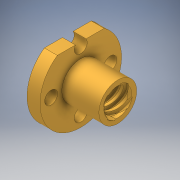
# Autodesk Inventor part: T8_Lead_Screw_Nut
Saved by Autodesk Inventor 2020.3 (Build 243373000, 373)
## iProperties
Created: 2020-06-14
Part Number: T8_Lead_Screw_Nut
Material: Brass, Soft Yellow
Document SubType Name: Modeling
Designer: rah75
Density: 8.47 g/cm^3
Appearance: Brass - Satin
Author: rah75
Autodesk Inventor part; units mm, degrees
ref_plane "YZ Plane" through (0, 0, 0) normal (1, 0, 0) x (0, 1, 0)
ref_plane "XZ Plane" through (0, 0, 0) normal (0, 1, 0) x (-1, 0, 0)
ref_plane "XY Plane" through (0, 0, 0) normal (0, 0, 1) x (1, 0, 0)
sketch "Sketch1" plane through (0, 0, 0) normal (0, 0, 1) x (1, 0, 0)
  line L0 (-1.75, 3.25) -> (11.75, 3.25)
  line L1 (11.75, 3.25) -> (11.75, 5.1)
  line L2 (11.75, 5.1) -> (1.75, 5.1)
  line L3 (1.75, 5.1) -> (1.75, 11)
  line L4 (1.75, 11) -> (-1.75, 11)
  line L5 (-1.75, 11) -> (-1.75, 3.25)
  line L6 (0, 0) -> (3.0338, 0)
  line L7 (-1.75, 5.1) -> (-3.25, 5.1)
  line L8 (-3.25, 5.1) -> (-3.25, 3.25)
  line L9 (-3.25, 3.25) -> (-1.75, 3.25)
  point P0 (0, 11)
  dimension "d2" = 10.2
  dimension "d3" = 6.5
  dimension "d4" = 22
  dimension "d5" = 3.5
  dimension "d6" = 10
  dimension "d7" = 1.5
  constraints: 20 end point, 7 perpendicular, 3 horizontal, 1 collinear, 1 midpoint, 1 point on line, 1 vertical alignment
  measures "d2" diameter of L2 L6
  measures "d3" diameter of L0 L6
  measures "d4" diameter of L4 L6
  measures "d5" distance of L3.end L4.end
  measures "d6" distance of L1.end L2.end
  measures "d7" distance of L7.start L7.end
revolve "Revolution1" add sketch "Sketch1" angle 360 about axis through (0, 0, 0) along (1, 0, 0)
sketch "Sketch2" plane through (0, 0, 0) normal (0, 0, 1) x (1, 0, 0)
  line L0 (11.75, 3.125) -> (13.018, 3.125)
  line L1 (13.018, 3.125) -> (12.75, 4)
  line L2 (12.75, 4) -> (12.018, 4)
  line L3 (12.018, 4) -> (11.75, 3.125)
  line L4 (11.75, -3.25) -> (11.75, 3.25) projected
  line L5 (11.75, 0) -> (12.6787, 0)
  line L6 (12.75, 4) -> (13.2458, 4) construction
  line L7 (12.018, 4) -> (11.5222, 4) construction
  line L8 (11.75, -5.1) -> (11.75, 5.1) projected
  line L9 (13.018, 3.125) -> (13.384, 3.125)
  line L10 (11.75, 3.125) -> (11.384, 3.125)
  point P0 (0, 0)
  dimension "d9" = 8
  dimension "d10" = 6.25
  dimension "d22" = 0.732
  dimension "d23" = 0.366
  dimension "d24" = 2
  constraints: 18 end point, 4 horizontal, 3 equal length, 3 point on line, 1 midpoint, 1 parallel
  measures "d9" diameter of L2 L5
  measures "d10" diameter of L0 L5
  measures "d22" distance of L1.end L2.end
  measures "d23" distance of L0.start L10.end
  measures "d24" distance of L9.end L10.end
coil "Coil1" sketch "Sketch2" operation cut axis through (11.75, 0, 0) along (-1, 0, 0) pitch 8 turns 2.5 hand right
chamfer "Chamfer1" distance 0.5 angle 45 3 edges at (-3.25, -3.1166, -0.9214) (11.75, 3.2496, -0.0489) (11.75, -2.8784, 1.5092)
sketch "Sketch3" plane through (1.75, 0, 0) normal (1, 0, 0) x (0, 0, -1)
  circle A0 centre (-8, 0) radius 1.75
  point P0 (0, 0)
  dimension "d31" = 8
  dimension "d32" = 3.5
  constraints: 1 centre point, 1 horizontal alignment
  measures "d31" distance of A0.centre point (0, 0)
  measures "d32" diameter of A0
extrude "Extrusion1" cut sketch "Sketch3" against normal blind 10
pattern_circular "Circular Pattern1" count 4 over 360 about axis through (4.25, 0, 0) along (1, 0, 0) of "Coil1", "Extrusion1"
sketch "Sketch4" plane through (-1.75, 0, 0) normal (-1, 0, 0) x (0, 0, 1)
  point P0 (0, 0)
sketch "Sketch5" plane through (-1.75, 0, 0) normal (-1, 0, 0) x (0, 0, 1)
  circle A0 centre (0, 0) radius 11 projected
  line L0 (-6.3246, 9) -> (6.3246, 9)
  circle A1 centre (0, 8) radius 1.75 projected
  circle A2 centre (8, 0) radius 1.75 projected
  line L1 (6.3246, 9) -> (8, 0) construction
  dimension "d35" = 9
  constraints: 4 end point, 2 point on circle, 1 horizontal
  measures "d35" distance from line of L0 point (0, 0)
extrude "Extrusion2" cut sketch "Sketch5" against normal blind 10 contours L0 A1 A0 | L0 A1 picked at (3.9044, 9.4218) picked at (0.3855, 9.1045)
equation "\"d23\" = 0.5 * d22"
body "Solid1"
